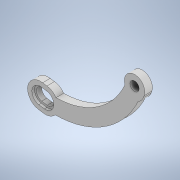
# Autodesk Inventor part: Part7
Saved by Autodesk Inventor 2020.3 (Build 243373000, 373)
## iProperties
Created: 2019-09-27
Part Number: Part7
Material: Generic
Document SubType Name: Modeling
Designer: Horváth Patrik
Density: 1 g/cm^3
Appearance: Default
Author: Horváth Patrik
Autodesk Inventor part; units mm, degrees
note: some values were not read from the file. Chosen so that the rebuilt part matches the saved one: second side of "Extrusion3".
ref_plane "YZ Plane" through (0, 0, 0) normal (1, 0, 0) x (0, 1, 0)
ref_plane "XZ Plane" through (0, 0, 0) normal (0, 1, 0) x (-1, 0, 0)
ref_plane "XY Plane" through (0, 0, 0) normal (0, 0, 1) x (1, 0, 0)
sketch "Sketch1" plane through (0, 0, 0) normal (0, 0, 1) x (1, 0, 0)
  circle A0 centre (36, 22) radius 1.25
  circle A1 centre (36, 22) radius 3
  arc A2 (0, 0) -> (36, 22) centre (4.7671, 32.6539) ccw construction
  arc A3 (-0.4334, -2.9685) -> (38.8394, 21.0315) centre (4.7671, 32.6539) ccw
  arc A4 (0.4334, 2.9685) -> (33.1606, 22.9685) centre (4.7671, 32.6539) ccw
  arc A5 (0.4334, 2.9685) -> (-0.4334, -2.9685) centre (0, 0) ccw
  arc A6 (38.8394, 21.0315) -> (33.1606, 22.9685) centre (36, 22) ccw
  point P0 (41.5332, 21.1583)
  point P1 (35.8668, 23.1312)
  point P2 (38.8394, 21.0315)
  point P3 (33.1606, 22.9685)
  dimension "d1" = 30
  dimension "d21" = 6
  dimension "d22" = 2.5
  dimension "d23" = 36
  dimension "d24" = 22
  constraints: 10 point on circle, 7 centre point, 4 tangent, 2 coincident, 1 concentric
  measures "d1" radius of A4
  measures "d21" radial gap between concentric circles of A3 A4
  measures "d22" diameter of A0
  measures "d23" horizontal distance of point (0, 0) A0.centre
  measures "d24" vertical distance of point (0, 0) A0.centre
extrude "Extrusion1" add sketch "Sketch1" along normal blind 3
sketch "Sketch3" plane through (0, 0, 3) normal (0, 0, 1) x (1, 0, 0)
  arc A0 (-1, 0.1617) -> (1, -0.1304) centre (4.7671, 32.6539) ccw construction
  arc A1 (-1.8738, -4.7614) -> (0.4292, -5.0977) centre (4.7671, 32.6539) ccw
  arc A2 (-0.1262, 5.0848) -> (1.5708, 4.8369) centre (4.7671, 32.6539) ccw
  arc A3 (-0.1262, 5.0848) -> (-1.8738, -4.7614) centre (-1, 0.1617) ccw
  arc A4 (0.4292, -5.0977) -> (1.5708, 4.8369) centre (1, -0.1304) ccw
  arc A5 (-0.4334, -2.9685) -> (38.8394, 21.0315) centre (4.7671, 32.6539) ccw projected
  point P0 (0, 0)
  dimension "d31" = 10
  dimension "d32" = 1
  dimension "d33" = 1
  constraints: 11 point on circle, 5 centre point, 4 tangent, 1 concentric
  measures "d31" radial gap between concentric circles of A1 A2
  measures "d32" horizontal distance of point (0, 0) A0.start
  measures "d33" horizontal distance of A0.end point (0, 0)
extrude "Extrusion3" add sketch "Sketch3" against normal blind 3
sketch "Sketch4" plane through (0, 0, 3) normal (0, 0, -1) x (1, 0, 0)
  arc A0 (-1.8738, 4.7614) -> (-0.1262, -5.0848) centre (-1, -0.1617) ccw projected
  arc A1 (0.4292, 5.0977) -> (-1.8738, 4.7614) centre (4.7671, -32.6539) ccw projected
  arc A2 (1.5708, -4.8369) -> (-0.1262, -5.0848) centre (4.7671, -32.6539) ccw projected
  arc A3 (1, 0.1304) -> (-1, -0.1617) centre (4.7671, -32.6539) ccw construction
  arc A4 (0.7146, 2.6141) -> (-1.4369, 2.2998) centre (4.7671, -32.6539) ccw
  arc A5 (1.2854, -2.3532) -> (-0.5631, -2.6232) centre (4.7671, -32.6539) ccw
  arc A6 (1.2854, -2.3532) -> (0.7146, 2.6141) centre (1, 0.1304) ccw
  arc A7 (-1.4369, 2.2998) -> (-0.5631, -2.6232) centre (-1, -0.1617) ccw
  arc A8 (33.1606, -22.9685) -> (5.1514, -2.6563) centre (4.7671, -32.6539) ccw projected
  arc A9 (33.1606, -22.9685) -> (38.8394, -21.0315) centre (36, -22) ccw projected
  arc A10 (38.8394, -21.0315) -> (4.8288, 3.3461) centre (4.7671, -32.6539) ccw projected
  arc A11 (4.8288, 3.3461) -> (0.4292, 5.0977) centre (1, 0.1304) ccw projected
  arc A12 (1.5708, -4.8369) -> (5.1514, -2.6563) centre (1, 0.1304) ccw projected
  arc A13 (1.3767, -3.148) -> (-0.4233, -3.4109) centre (4.7671, -32.6539) ccw
  arc A14 (1.3767, -3.148) -> (0.6233, 3.4088) centre (1, 0.1304) ccw
  arc A15 (0.6233, 3.4088) -> (-1.5767, 3.0875) centre (4.7671, -32.6539) ccw
  arc A16 (-1.5767, 3.0875) -> (-0.4233, -3.4109) centre (-1, -0.1617) ccw
  point P0 (0, 0)
  dimension "d43" = 5
  dimension "d52" = 0.8
  constraints: 18 point on circle, 9 centre point, 4 tangent, 2 coincident, 1 concentric, 3 other
  measures "d43" radial gap between concentric circles of A4 A5
  measures "d52" radial gap between concentric circles of A5 A13
extrude "Extrusion4" cut sketch "Sketch4" along normal through all contours A6 A5 A7 A4
sketch "Sketch5" plane through (0, 0, 3) normal (0, 0, 1) x (1, 0, 0)
  circle A0 centre (36, 22) radius 1.25 projected
  arc A1 (0, 0) -> (36, 22) centre (4.7671, 32.6539) ccw construction
  arc A2 (39.7686, 20.6592) -> (32.2314, 23.3408) centre (36, 22) ccw
  arc A3 (31.9418, 22.5269) -> (39.479, 19.8452) centre (35.7104, 21.1861) ccw
  line L0 (35.0504, 21.4307) -> (36.2779, 20.9758)
  line L1 (37.5646, 21.4663) -> (34.5144, 22.5068)
  line L2 (31.9418, 22.5269) -> (32.2314, 23.3408)
  line L3 (39.479, 19.8452) -> (39.7686, 20.6592)
  circle A4 centre (36, 22) radius 1.8
  dimension "d44" = 8
  dimension "d46" = 1.5
  dimension "d47" = 3.6
  constraints: 8 end point, 5 point on circle, 4 tangent, 3 centre point, 2 coincident, 2 line through centre, 2 point on line, 1 equal radius
  measures "d44" diameter of A2
  measures "d46" angle of L1 L0
  measures "d47" diameter of A4
extrude "Extrusion5" cut sketch "Sketch5" against normal up to surface (3 mm away) contours A4
extrude "Extrusion6" add sketch "Sketch5" against normal up to surface (3 mm away) contours L3 A3 L2 A2
extrude "Extrusion7" cut sketch "Sketch4" along normal blind 1 contours A13 A16 A15 A14
sketch "Sketch6" plane through (0, 0, 0) normal (0, 0, -1) x (-1, 0, 0)
  circle A0 centre (-36, 22) radius 1.8 projected
  arc A1 (-37.4644, 17.5911) -> (-4.8288, -3.3461) centre (-4.7671, 32.6539) ccw projected
  arc A2 (-4.8288, -3.3461) -> (-0.4292, -5.0977) centre (-1, -0.1304) ccw projected
  arc A3 (-0.4292, -5.0977) -> (1.8738, -4.7614) centre (-4.7671, 32.6539) ccw projected
  arc A4 (1.8738, -4.7614) -> (0.1262, 5.0848) centre (1, 0.1617) ccw projected
  arc A5 (-1.5708, 4.8369) -> (0.1262, 5.0848) centre (-4.7671, 32.6539) ccw projected
  arc A6 (-1.5708, 4.8369) -> (-5.1514, 2.6563) centre (-1, -0.1304) ccw projected
  arc A7 (-31.9221, 19.9021) -> (-5.1514, 2.6563) centre (-4.7671, 32.6539) ccw projected
  arc A8 (-31.9221, 19.9021) -> (-31.9418, 22.5269) centre (-35.7104, 21.1861) ccw projected
  line L0 (-31.9418, 22.5269) -> (-32.2314, 23.3408) projected
  arc A9 (-32.2314, 23.3408) -> (-39.7686, 20.6592) centre (-36, 22) ccw projected
  line L1 (-39.7686, 20.6592) -> (-39.479, 19.8452) projected
  arc A10 (-39.479, 19.8452) -> (-37.4644, 17.5911) centre (-35.7104, 21.1861) ccw projected
  arc A11 (-0.7146, -2.6141) -> (1.4369, -2.2998) centre (-4.7671, 32.6539) ccw projected
  arc A12 (-1.2854, 2.3532) -> (-0.7146, -2.6141) centre (-1, -0.1304) ccw projected
  arc A13 (-1.2854, 2.3532) -> (0.5631, 2.6232) centre (-4.7671, 32.6539) ccw projected
  arc A14 (1.4369, -2.2998) -> (0.5631, 2.6232) centre (1, 0.1617) ccw projected
  arc A15 (-32.2314, 23.3408) -> (-39.7686, 20.6592) centre (-36, 22) ccw projected
  arc A16 (-32.2466, 20.6173) -> (-32.2314, 23.3408) centre (-36, 22) ccw
  arc A17 (-31.9221, 19.9021) -> (-5.1514, 2.6563) centre (-4.7671, 32.6539) ccw projected
  arc A18 (-32.2466, 20.6173) -> (-31.9221, 19.9021) centre (-4.7671, 32.6539) ccw
  arc A19 (-31.9221, 19.9021) -> (-5.1514, 2.6563) centre (-4.7671, 32.6539) ccw projected
  point P0 (0, 0)
  constraints: 6 point on circle, 3 concentric, 2 centre point
extrude "Extrusion8" cut sketch "Sketch6" against normal up to surface (3 mm away) contours L0 A8 A18 A16
body "Solid1"
